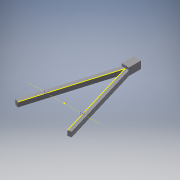
# Autodesk Inventor part: deichsel
Saved by Autodesk Inventor 2018 (Build 220112000, 112)
## iProperties
Created: 2020-03-25
Part Number: deichsel
Material: Generisch
Document SubType Name: Blech
Designer: wepet
Density: 1 g/cm^3
Sheet Metal Rule: Standard_mm
Appearance: Vorgabe
Author: wepet
Autodesk Inventor part; units mm, degrees
ref_plane "YZ Plane" through (0, 0, 0) normal (1, 0, 0) x (0, 1, 0)
ref_plane "XZ Plane" through (0, 0, 0) normal (0, 1, 0) x (-1, 0, 0)
ref_plane "XY Plane" through (0, 0, 0) normal (0, 0, 1) x (1, 0, 0)
sketch "Skizze1" plane through (0, 0, 0) normal (0, 0, 1) x (1, 0, 0)
  line L0 (-75, 0) -> (75, 0) construction
  circle A0 centre (0, 0) radius 37.5 construction
  line L1 (0, 0) -> (0, 125) construction
  line L2 (0, 125) -> (0, 150) construction
  line L3 (-7.5, 150) -> (7.5, 150) construction
  line L4 (-7.5, 125) -> (7.5, 125) construction
  line L5 (-7.5, 150) -> (7.5, 150)
  line L6 (7.5, 125) -> (7.5, 150)
  line L7 (-7.5, 150) -> (-7.5, 125)
  circle A1 centre (0, 0) radius 45 construction
  line L8 (-7.5, 125) -> (-57.7859, -42.6196)
  line L9 (7.5, 125) -> (57.7859, -42.6196)
  line L10 (-50.6022, -44.7747) -> (0, 123.8992)
  line L11 (0, 123.8992) -> (50.6022, -44.7747)
  line L12 (-57.7859, -42.6196) -> (-50.6022, -44.7747)
  line L13 (57.7859, -42.6196) -> (50.6022, -44.7747)
  point P0 (-45, 0)
  point P1 (45, 0)
  dimension "d0" = 150
  dimension "d1" = 75
  dimension "d2" = 125
  dimension "d3" = 25
  dimension "d4" = 15
  dimension "d5" = 90
  dimension "d6" = 175
  dimension "d7" = 175
  dimension "d8" = 7.5
  dimension "d9" = 7.5
  constraints: 28 end point, 5 point on line, 4 perpendicular, 3 coincident, 3 horizontal, 3 midpoint, 2 centre point, 2 parallel, 2 point on circle, 1 collinear, 1 vertical
  measures "d0" distance of L0.start L0.end
  measures "d1" diameter of A0
  measures "d2" distance of L1.end L1.start
  measures "d3" distance of L2.end L1.end
  measures "d4" distance of L3.start L3.end
  measures "d5" diameter of A1
  measures "d6" distance of L4.start L8.end
  measures "d7" distance of L4.end L9.end
  measures "d8" distance between parallel lines of L8 L10
  measures "d9" distance between parallel lines of L9 L11
extrude "Extrusion1" add sketch "Skizze1" along normal blind 10
sketch "Skizze2" plane through (0, 0, 10) normal (0, 0, 1) x (1, 0, 0)
  line L0 (-7.5, 150) -> (-7.5, 125) projected
  line L1 (7.5, 150) -> (-7.5, 150) projected
  line L2 (7.5, 125) -> (7.5, 150) projected
  line L3 (-7.5, 125) -> (7.5, 125)
  point P0 (0, 0)
  constraints: 2 end point, 1 horizontal
extrude "Extrusion2" add sketch "Skizze2" along normal blind 5
sketch "Skizze3" plane through (0, 0, 10) normal (0, 0, 1) x (1, 0, 0)
  line L0 (-75, 0) -> (75, 0) construction
  line L1 (-50.6022, -44.7747) -> (0, 123.8992) projected
  line L2 (0, 123.8992) -> (50.6022, -44.7747) projected
  point P0 (0, 0)
  point P1 (-37.1698, 0)
  point P2 (37.1698, 0)
  constraints: 4 point on line
equation "\"Biegeradius\" = Stärke"
equation "\"BreiteBiegungsfreistellung\" = Stärke"
equation "\"TiefeBiegungsfreistellung\" = 0.5 * Stärke"
equation "\"GrößeEckenfreistellung\" = 4 * Stärke"
equation "\"MinimalRest\" = 2 * Stärke"
equation "\"Übergangsradius\" = Biegeradius"
equation "\"JacobiRadiusGröße\" = Biegeradius"
equation "\"Abstandsgröße\" = Stärke"
equation "\"Stärke\" = 0.5"
